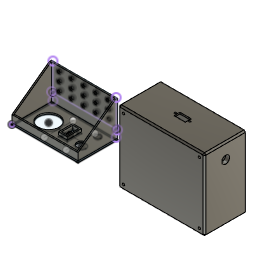
12v-socket-mounting-bracket_and_case (Autodesk Fusion 360 design; units mm, degrees)
Autodesk Fusion 360 part; units mm, degrees
sketch "Skizze1" plane through (0, 0, 0) normal (0, 0, 1) x (1, 0, 0) in component "Montagewinkel"
  line L0 (0, 0) -> (92, 0)
  line L1 (92, 0) -> (92, 55)
  line L2 (92, 55) -> (0, 55)
  line L3 (0, 55) -> (0, 0)
  line L4 (2, 2) -> (90, 2)
  line L5 (90, 2) -> (90, 53)
  line L6 (90, 53) -> (2, 53)
  line L7 (2, 53) -> (2, 2)
  line L8 (2, 53) -> (2, 55)
  line L9 (90, 53) -> (90, 55)
  line L10 (2, 2) -> (2, 0)
  line L11 (90, 2) -> (90, 0)
  circle A0 centre (23.5, 27.5) radius 14.5
  circle A1 centre (74.5, 22) radius 6
  circle A2 centre (74.5, 45) radius 4
  line L12 (38, 47) -> (38, 7) construction
  line L13 (68.5, 47) -> (68.5, 7) construction
  line L14 (68.5, 27.5) -> (38, 27.5) construction
  line L15 (57.325, 19.625) -> (49.175, 19.625)
  line L16 (49.175, 19.625) -> (49.175, 35.375)
  line L17 (49.175, 35.375) -> (57.325, 35.375)
  line L18 (57.325, 35.375) -> (57.325, 19.625)
  line L19 (57.325, 19.625) -> (49.175, 35.375) construction
  line L20 (49.175, 19.625) -> (57.325, 35.375) construction
  line L21 (59.325, 17.625) -> (47.175, 17.625)
  line L22 (47.175, 17.625) -> (47.175, 37.375)
  line L23 (47.175, 37.375) -> (59.325, 37.375)
  line L24 (59.325, 37.375) -> (59.325, 17.625)
  point P0 (53.25, 27.5)
  dimension "d1" = 92
  dimension "d2" = 55
  dimension "d4" = 29
  dimension "d5" = 23.5
  dimension "d6" = 27.5
  dimension "d7" = 12
  dimension "d8" = 22
  dimension "d9" = 17.5
  dimension "d10" = 8
  dimension "d11" = 10
  dimension "d12" = 17.5
  dimension "d13" = 27.5
  dimension "d14" = 8.15
  dimension "d15" = 15.75
  constraint horizontal L0
  constraint vertical L1
  constraint horizontal L2
  constraint vertical L3
  constraint coincident L0.start L3.end
  constraint coincident L2 L8.end
  constraint perpendicular L2 L8
  constraint coincident L2 L9.end
  constraint perpendicular L2 L9
  constraint coincident L0 L10.end
  constraint perpendicular L0 L10
  constraint coincident L0 L11.end
  constraint perpendicular L0 L11
  constraint vertical L12
  constraint tangent A0 L12
  constraint vertical L13
  constraint tangent A1 L13
  constraint coincident L13 L14.start
  constraint coincident L12 L14.end
  constraint perpendicular L12 L14
  constraint horizontal L15
  constraint perpendicular L15 L16
  constraint parallel L15 L17
  constraint parallel L16 L18
  constraint coincident L19 P0
  constraint coincident L20 P0
  constraint midpoint L14 P0
  measures "d1" distance of L0.start L0.end
  measures "d2" distance of L0.start L2.end
  measures "d4" diameter of A0
  measures "d5" distance of L3 A0.centre
  measures "d6" distance of L2 A0.centre
  measures "d7" diameter of A1
  measures "d8" distance of L0 A1.centre
  measures "d9" distance of L1 A1.centre
  measures "d10" diameter of A2
  measures "d11" distance of L2 A2.centre
  measures "d12" distance of L1 A2.centre
  measures "d13" distance of L2 L14
  measures "d14" distance of L16.end L17.end
  measures "d15" distance of L15.end L16.end
extrude "Extrusion1" add sketch "Skizze1" along normal blind 2 contours L4 L5 L6 L7 makes body 1 in component "Montagewinkel"
extrude "Extrusion3" add sketch "Skizze1" along normal blind 6 contours L21 L22 L23 L24 bodies 1 in component "Montagewinkel"
extrude "Extrusion4" add sketch "Skizze1" along normal blind 50 contours L0 L2 L3 L7 L8 L10 | L0 L1 L2 L5 L9 L11 | L2 L6 L8 L9 bodies 1 in component "Montagewinkel"
extrude "Extrusion5" add sketch "Skizze1" along normal blind 12 contours L0 L4 L10 L11 bodies 1 in component "Montagewinkel"
chamfer "Fase1" distance 52 distance2 38 2 edges at (1, 0, 50) (91, 0, 50) measured on face at (31.3333, 54.3333, 50) measured on face at (31.3333, 54.3333, 50) on bodies 1 in component "Montagewinkel"
chamfer "Fase2" distance 2 angle 45 3 edges at (46, 0, 0) (0, 27.5, 0) (92, 27.5, 0) on bodies 1 in component "Montagewinkel"
sketch "Skizze2" plane through (0, 55, 0) normal (0, 1, 0) x (-1, 0, 0) in component "Montagewinkel"
  line L0 (-92, 2) -> (-90, 0)
  line L1 (-90, 0) -> (-2, 0)
  line L2 (-2, 0) -> (0, 2)
  line L3 (0, 2) -> (0, 50)
  line L4 (0, 50) -> (-92, 50)
  line L5 (-92, 50) -> (-92, 2)
  line L6 (0, 12) -> (-2, 12)
  line L7 (-2, 12) -> (-90, 12)
  line L8 (-90, 12) -> (-92, 12)
  line L9 (-2, 2) -> (-2, 50)
  line L10 (-90, 2) -> (-90, 50)
  circle A0 centre (-80, 19) radius 1.8
  circle A1 centre (-63, 19) radius 1.8
  circle A2 centre (-80, 31) radius 1.8
  circle A3 centre (-63, 31) radius 1.8
  circle A4 centre (-46, 19) radius 1.8
  circle A5 centre (-29, 19) radius 1.8
  circle A6 centre (-12, 19) radius 1.8
  circle A7 centre (-46, 31) radius 1.8
  circle A8 centre (-29, 31) radius 1.8
  circle A9 centre (-12, 31) radius 1.8
  circle A10 centre (-80, 43) radius 1.8
  circle A11 centre (-63, 43) radius 1.8
  circle A12 centre (-46, 43) radius 1.8
  circle A13 centre (-29, 43) radius 1.8
  circle A14 centre (-12, 43) radius 1.8
  dimension "d30" = 3.6
  dimension "d31" = 10
  dimension "d32" = 7
  dimension "d36" = 68
  dimension "d37" = 24
  measures "d30" diameter of A0
  measures "d31" distance of L10 A0.centre
  measures "d32" distance of L7 A0.centre
extrude "Extrusion6" cut sketch "Skizze2" against normal blind 2 contours A0 | A1 | A2 | A3 | A4 | A5 | A6 | A7 | A8 | A9 | A10 | A11 | A12 | A13 | A14 bodies 1 in component "Montagewinkel"
sketch "Skizze1 (2)" plane through (0, 0, 0) normal (0, 0, 1) x (1, 0, 0) in component "Gehäuse"
  line L0 (0, 0) -> (120, 0)
  line L1 (120, 0) -> (120, 55)
  line L2 (120, 55) -> (0, 55)
  line L3 (0, 55) -> (0, 0)
  circle A0 centre (32.7, 27.5) radius 14.5
  circle A1 centre (93.3, 22) radius 6
  circle A2 centre (93.3, 45) radius 4
  line L4 (47.2, 47) -> (47.2, 7) construction
  line L5 (87.3, 47) -> (87.3, 7) construction
  line L6 (87.3, 27.5) -> (47.2, 27.5) construction
  line L7 (71.325, 19.625) -> (63.175, 19.625)
  line L8 (63.175, 19.625) -> (63.175, 35.375)
  line L9 (63.175, 35.375) -> (71.325, 35.375)
  line L10 (71.325, 35.375) -> (71.325, 19.625)
  line L11 (71.325, 19.625) -> (63.175, 35.375) construction
  line L12 (63.175, 19.625) -> (71.325, 35.375) construction
  line L13 (73.325, 17.625) -> (61.175, 17.625)
  line L14 (61.175, 17.625) -> (61.175, 37.375)
  line L15 (61.175, 37.375) -> (73.325, 37.375)
  line L16 (73.325, 37.375) -> (73.325, 17.625)
  point P0 (67.25, 27.5)
  dimension "d1_1" = 120
  dimension "d2_1" = 55
  dimension "d4_1" = 29
  dimension "d5_1" = 32.7
  dimension "d6_1" = 27.5
  dimension "d7_1" = 12
  dimension "d8_1" = 22
  dimension "d9_1" = 26.7
  dimension "d10_1" = 8
  dimension "d11_1" = 10
  dimension "d12_1" = 26.7
  dimension "d13_1" = 27.5
  dimension "d14_1" = 8.15
  dimension "d15_1" = 15.75
  constraint horizontal L0
  constraint vertical L1
  constraint horizontal L2
  constraint vertical L3
  constraint coincident L0.start L3.end
  constraint vertical L4
  constraint tangent A0 L4
  constraint vertical L5
  constraint tangent A1 L5
  constraint coincident L5 L6.start
  constraint coincident L4 L6.end
  constraint perpendicular L4 L6
  constraint horizontal L7
  constraint perpendicular L7 L8
  constraint parallel L7 L9
  constraint parallel L8 L10
  constraint coincident L11 P0
  constraint coincident L12 P0
  constraint midpoint L6 P0
  measures "d1_1" distance of L0.start L0.end
  measures "d2_1" distance of L0.start L2.end
  measures "d4_1" diameter of A0
  measures "d5_1" distance of L3 A0.centre
  measures "d6_1" distance of L2 A0.centre
  measures "d7_1" diameter of A1
  measures "d8_1" distance of L0 A1.centre
  measures "d9_1" distance of L1 A1.centre
  measures "d10_1" diameter of A2
  measures "d11_1" distance of L2 A2.centre
  measures "d12_1" distance of L1 A2.centre
  measures "d13_1" distance of L2 L6
  measures "d14_1" distance of L8.end L9.end
  measures "d15_1" distance of L7.end L8.end
extrude "Extrusion8" add sketch "Skizze1 (2)" along normal blind 100 separate body contours L0 L1 L2 L3 | A0 | A1 | A2 | L7 L8 L9 L10 | L13 L14 L15 L16 makes body 2 in component "Gehäuse"
shell "Schale1" thickness 2 removed faces 1 at (40, 0, 66.6667) on bodies 2 in component "Gehäuse"
chamfer "Fase4" distance 2 angle 45 4 edges at (120, 27.5, 100) (0, 27.5, 100) (0, 27.5, 0) (120, 27.5, 0) on bodies 2 in component "Gehäuse"
extrude "Extrusion9" cut sketch "Skizze1 (2)" along normal blind 2 contours A0 | A1 | A2 | L7 L8 L9 L10 bodies 2 in component "Gehäuse"
extrude "Extrusion10" add sketch "Skizze1 (2)" along normal blind 6 contours L13 L14 L15 L16 bodies 2 in component "Gehäuse"
sketch "Skizze4" plane through (0, 53, 0) normal (0, -1, 0) x (1, 0, 0) in component "Gehäuse"
  line L0 (2, 2) -> (118, 2)
  line L1 (118, 2) -> (118, 98)
  line L2 (118, 98) -> (2, 98)
  line L3 (2, 98) -> (2, 2)
  circle A0 centre (7.2, 92.8) radius 5.2
  circle A1 centre (7.2, 92.8) radius 1.25
  circle A2 centre (112.8, 92.8) radius 5.2
  circle A3 centre (112.8, 92.8) radius 1.25
  circle A4 centre (7.2, 7.2) radius 5.2
  circle A5 centre (7.2, 7.2) radius 1.25
  circle A6 centre (112.8, 7.2) radius 5.2
  circle A7 centre (112.8, 7.2) radius 1.25
  line L4 (12.4, 92.8) -> (12.4, 98)
  line L5 (7.2, 87.6) -> (2, 87.6)
  line L6 (107.6, 92.8) -> (107.6, 98)
  line L7 (112.8, 87.6) -> (118, 87.6)
  line L8 (12.4, 7.2) -> (12.4, 2)
  line L9 (7.2, 12.4) -> (2, 12.4)
  line L10 (112.8, 12.4) -> (118, 12.4)
  line L11 (107.6, 7.2) -> (107.6, 2)
  line L12 (13.5, 62) -> (7, 62)
  line L13 (7, 62) -> (7, 77)
  line L14 (7, 77) -> (13.5, 77)
  line L15 (13.5, 77) -> (13.5, 62)
  line L16 (13.5, 62) -> (7, 77) construction
  line L17 (7, 62) -> (13.5, 77) construction
  line L18 (55, 62) -> (48.5, 62)
  line L19 (48.5, 62) -> (48.5, 77)
  line L20 (48.5, 77) -> (55, 77)
  line L21 (55, 77) -> (55, 62)
  line L22 (55, 62) -> (48.5, 77) construction
  line L23 (48.5, 62) -> (55, 77) construction
  line L24 (113, 42) -> (106.5, 42)
  line L25 (106.5, 42) -> (106.5, 57)
  line L26 (106.5, 57) -> (113, 57)
  line L27 (113, 57) -> (113, 42)
  line L28 (113, 42) -> (106.5, 57) construction
  line L29 (106.5, 42) -> (113, 57) construction
  line L30 (71.5, 42) -> (65, 42)
  line L31 (65, 42) -> (65, 57)
  line L32 (65, 57) -> (71.5, 57)
  line L33 (71.5, 57) -> (71.5, 42)
  line L34 (71.5, 42) -> (65, 57) construction
  line L35 (65, 42) -> (71.5, 57) construction
  circle A8 centre (10.25, 69.5) radius 1.25
  circle A9 centre (68.25, 49.5) radius 1.25
  circle A10 centre (51.75, 69.5) radius 1.25
  circle A11 centre (109.75, 49.5) radius 1.25
  circle A12 centre (12, 22) radius 1.8
  line L36 (60, 98) -> (60, 2) construction
  circle A13 centre (108, 22) radius 1.8
  circle A14 centre (22, 88) radius 1.8
  line L37 (2, 98) -> (118, 98)
  line L38 (2, 2) -> (2, 98)
  circle A15 centre (98, 88) radius 1.8
  line L39 (118, 98) -> (118, 2)
  point P0 (10.25, 69.5)
  point P1 (51.75, 69.5)
  point P2 (109.75, 49.5)
  point P3 (68.25, 49.5)
  dimension "d68" = 5.2
  dimension "d69" = 2.5
  dimension "d70" = 5.2
  dimension "d71" = 2.5
  dimension "d72" = 5.2
  dimension "d73" = 2.5
  dimension "d74" = 5.2
  dimension "d75" = 2.5
  dimension "d78" = 6.5
  dimension "d79" = 15
  dimension "d80" = 5
  dimension "d81" = 60
  dimension "d82" = 15
  dimension "d83" = 6.5
  dimension "d84" = 48
  dimension "d85" = 60
  dimension "d86" = 15
  dimension "d87" = 6.5
  dimension "d88" = 5
  dimension "d89" = 6.5
  dimension "d90" = 15
  dimension "d91" = 48
  dimension "d92" = 40
  dimension "d93" = 40
  dimension "d94" = 2.5
  dimension "d95" = 2.5
  dimension "d96" = 2.5
  dimension "d97" = 2.5
  dimension "d162" = 3.6
  dimension "d163" = 20
  dimension "d164" = 10
  dimension "d165" = 3.6
  dimension "d166" = 10
  dimension "d167" = 20
  dimension "d168" = 3.6
  dimension "d169" = 10
  dimension "d170" = 20
  constraint tangent L2 A0
  constraint tangent L3 A0
  constraint concentric A0 A1
  constraint tangent L2 A2
  constraint tangent L1 A2
  constraint concentric A2 A3
  constraint tangent L3 A4
  constraint tangent L0 A4
  constraint concentric A4 A5
  constraint tangent L0 A6
  constraint tangent L1 A6
  constraint concentric A6 A7
  constraint coincident A0 L4.start
  constraint coincident L2 L4.end
  constraint tangent A0 L4
  constraint perpendicular L2 L4
  constraint coincident A0 L5.start
  constraint coincident L3 L5.end
  constraint tangent A0 L5
  constraint perpendicular L3 L5
  constraint coincident A2 L6.start
  constraint coincident L2 L6.end
  constraint tangent A2 L6
  constraint perpendicular L2 L6
  constraint coincident A2 L7.start
  constraint tangent A2 L7
  constraint perpendicular L6 L7
  constraint coincident A4 L8.start
  constraint coincident L0 L8.end
  constraint tangent A4 L8
  constraint perpendicular L0 L8
  constraint coincident A4 L9.start
  constraint coincident L3 L9.end
  constraint tangent A4 L9
  constraint perpendicular L3 L9
  constraint coincident A6 L10.start
  constraint coincident L1 L10.end
  constraint tangent A6 L10
  constraint perpendicular L1 L10
  constraint coincident A6 L11.start
  constraint coincident L0 L11.end
  constraint tangent A6 L11
  constraint perpendicular L0 L11
  constraint horizontal L12
  constraint perpendicular L12 L13
  constraint parallel L12 L14
  constraint parallel L13 L15
  constraint coincident L16 P0
  constraint coincident L17 P0
  constraint horizontal L18
  constraint perpendicular L18 L19
  constraint parallel L18 L20
  constraint parallel L19 L21
  constraint coincident L22 P1
  constraint coincident L23 P1
  constraint horizontal L24
  constraint perpendicular L24 L25
  constraint parallel L24 L26
  constraint parallel L25 L27
  constraint coincident L28 P2
  constraint coincident L29 P2
  constraint horizontal L30
  constraint perpendicular L30 L31
  constraint parallel L30 L32
  constraint parallel L31 L33
  constraint coincident L34 P3
  constraint coincident L35 P3
  constraint coincident P0 A8.centre
  constraint coincident P3 A9.centre
  constraint coincident P1 A10.centre
  constraint coincident P2 A11.centre
  constraint coincident L1 L7.end
  constraint midpoint L2 L36.start
  constraint midpoint L0 L36.end
  constraint symmetric A12 L36 A13
  measures "d68" radius of A0
  measures "d69" diameter of A1
  measures "d70" radius of A2
  measures "d71" diameter of A3
  measures "d72" radius of A4
  measures "d73" diameter of A5
  measures "d74" radius of A6
  measures "d75" diameter of A7
  measures "d78" distance of L13.end L14.end
  measures "d79" distance of L12.end L13.end
  measures "d80" distance of L3 L13
  measures "d81" distance of L0 L12
  measures "d82" distance of L18.end L19.end
  measures "d83" distance of L19.end L20.end
  measures "d84" distance of L13 L21
  measures "d85" distance of L0 L18
  measures "d86" distance of L24.end L25.end
  measures "d87" distance of L25.end L26.end
  measures "d88" distance of L1 L27
  measures "d89" distance of L31.end L32.end
  measures "d90" distance of L30.end L31.end
  measures "d91" distance of L27 L31
  measures "d92" distance of L0 L24
  measures "d93" distance of L0 L30
  measures "d94" diameter of A8
  measures "d95" diameter of A9
  measures "d96" diameter of A10
  measures "d97" diameter of A11
  measures "d162" diameter of A12
  measures "d163" distance of L0 A12.centre
  measures "d164" distance of L3 A12.centre
  measures "d165" diameter of A14
  measures "d166" distance of A14.centre L37
  measures "d167" distance of A14.centre L38
  measures "d168" diameter of A15
  measures "d169" distance of L2 A15.centre
  measures "d170" distance of A15.centre L39
extrude "Extrusion11" add sketch "Skizze4" along normal blind 53 contours L0 A4 L8 | L0 A6 L11 | L0 L3 A4 L38 | A4 | L0 L1 A6 L39 | A6 | L3 A4 L9 L38 | L1 A6 L10 L39 | L3 A0 L5 L38 | L1 A2 L7 L39 | L2 L3 A0 L37 L38 | A0 | L1 L2 A2 L37 L39 | A2 | L2 A0 L4 L37 | L2 A2 L6 L37 bodies 2 in component "Gehäuse"
extrude "Extrusion12" add sketch "Skizze4" along normal blind 15 contours L12 L13 L14 L15 | L18 L19 L20 L21 bodies 2 in component "Gehäuse"
extrude "Extrusion13" add sketch "Skizze4" along normal blind 20 contours L24 L25 L26 L27 | L30 L31 L32 L33 bodies 2 in component "Gehäuse"
extrude "Extrusion17" cut sketch "Skizze4" against normal blind 2 contours A12 | A13 | A14 | A15 bodies 2 in component "Gehäuse"
sketch "Skizze6" plane through (0, 0, 100) normal (0, 0, 1) x (-1, 0, 0) in component "Gehäuse"
  line L0 (-2, -55) -> (-2, 0)
  line L1 (-2, 0) -> (-118, 0)
  line L2 (-118, 0) -> (-118, -55)
  line L3 (-118, -55) -> (-2, -55)
  line L4 (-2, -55) -> (-118, 0) construction
  line L5 (-118, -55) -> (-2, 0) construction
  line L6 (-67.875, -23.425) -> (-52.125, -23.425)
  line L7 (-52.125, -23.425) -> (-52.125, -31.575)
  line L8 (-52.125, -31.575) -> (-67.875, -31.575)
  line L9 (-67.875, -31.575) -> (-67.875, -23.425)
  line L10 (-67.875, -23.425) -> (-52.125, -31.575) construction
  line L11 (-52.125, -23.425) -> (-67.875, -31.575) construction
  circle A0 centre (-49.75, -27.5) radius 1.25
  line L12 (-60, -31.575) -> (-60, -23.425) construction
  circle A1 centre (-70.25, -27.5) radius 1.25
  point P0 (-60, -27.5)
  dimension "d120" = 15.75
  dimension "d121" = 8.15
  dimension "d122" = 2.5
  dimension "d123" = 10.25
  dimension "d124" = 4.075
  constraint coincident L0.start L3.end
  constraint coincident L1.end L2.start
  constraint coincident L2.end L3.start
  constraint coincident L0.end L1.start
  constraint horizontal L6
  constraint perpendicular L6 L7
  constraint parallel L6 L8
  constraint parallel L7 L9
  constraint coincident L10 P0
  constraint coincident L11 P0
  constraint midpoint L4 P0
  constraint midpoint L8 L12.start
  constraint midpoint L6 L12.end
  constraint symmetric A0 L12 A1
  measures "d120" distance of L7.end L8.end
  measures "d121" distance of L6.end L7.end
  measures "d122" diameter of A0
  measures "d123" distance of P0 A0.centre
  measures "d124" distance of L6 A0.centre
extrude "Extrusion14" cut sketch "Skizze6" against normal blind 2 contours L6 L7 L8 L9 | A0 | A1 bodies 2 in component "Gehäuse"
sketch "Skizze7" plane through (120, 0, 0) normal (1, 0, 0) x (0, 1, 0) in component "Gehäuse"
  line L0 (0, 2) -> (55, 2)
  line L1 (55, 2) -> (55, 98)
  line L2 (55, 98) -> (0, 98)
  line L3 (0, 98) -> (0, 2)
  circle A0 centre (27.5, 78.8) radius 5.425
  line L4 (32.925, 73.375) -> (22.075, 73.375)
  line L5 (22.075, 73.375) -> (22.075, 84.225)
  line L6 (22.075, 84.225) -> (32.925, 84.225)
  line L7 (32.925, 84.225) -> (32.925, 73.375)
  line L8 (32.925, 73.375) -> (22.075, 84.225) construction
  line L9 (22.075, 73.375) -> (32.925, 84.225) construction
  line L10 (22.575, 84.225) -> (22.575, 73.375)
  circle A1 centre (27.5, 78.8) radius 7.425
  point P0 (27.5, 78.8)
  dimension "d148" = 10.85
  dimension "d149" = 27.5
  dimension "d150" = 19.2
  dimension "d151" = 10.85
  dimension "d152" = 10.85
  dimension "d153" = 4.925
  dimension "d158" = 2
  constraint horizontal L4
  constraint perpendicular L4 L5
  constraint parallel L4 L6
  constraint parallel L5 L7
  constraint coincident L8 P0
  constraint coincident L9 P0
  constraint coincident P0 A0.centre
  constraint coincident L6 L10.start
  constraint coincident L4 L10.end
  constraint perpendicular L4 L10
  measures "d148" diameter of A0
  measures "d149" distance of L1 P0
  measures "d150" distance of L2 P0
  measures "d151" distance of L5.end L6.end
  measures "d152" distance of L4.end L5.end
  measures "d153" distance of P0 L10
extrude "Extrusion15" cut sketch "Skizze7" against normal blind 2 contours A0 L10 picked at (25.8622, 77.1855) bodies 2 in component "Gehäuse"
extrude "Extrusion16" add sketch "Skizze7" against normal blind 5.5 contours A0 L4 L7 A1 | A0 L6 L7 A1 | L7 A1 | A0 L6 L10 | L6 A1 | A0 L4 L10 | L4 A1 | A0 L10 | A0 L5 L6 L10 A1 | A0 L4 L5 L10 A1 | L5 A1 picked at (22.4831, 79.3144) bodies 2 in component "Gehäuse"
draft "Entwurf5" angle 25 neutral plane through (0, 38, 0) pull (0, -1, 0) 1 faces at (55, 48, 72) on bodies 2 in component "Gehäuse"
draft "Entwurf6" angle 25 neutral plane through (0, 33, 0) pull (0, -1, 0) 1 faces at (65, 46.3333, 47) on bodies 2 in component "Gehäuse"
draft "Entwurf7" angle 25 neutral plane through (0, 38, 0) pull (0, -1, 0) 1 faces at (7, 48, 67) on bodies 2 in component "Gehäuse"
draft "Entwurf8" angle 25 neutral plane through (0, 33, 0) pull (0, -1, 0) 1 faces at (113, 46.3333, 52) on bodies 2 in component "Gehäuse"
sketch "Skizze1 (3)" plane through (0, 0, 0) normal (0, -1, 0) x (1, 0, 0) in component "Gehäusedeckel"
  circle A0 centre (262.8, 7.2) radius 1.25
  circle A1 centre (157.2, 92.8) radius 1.25
  circle A2 centre (157.2, 7.2) radius 1.25
  circle A3 centre (262.8, 92.8) radius 1.25
  line L0 (268, 0) -> (270, 2)
  line L1 (270, 2) -> (270, 98)
  line L2 (270, 98) -> (268, 100)
  line L3 (268, 100) -> (152, 100)
  line L4 (152, 100) -> (150, 98)
  line L5 (150, 98) -> (150, 2)
  line L6 (150, 2) -> (152, 0)
  line L7 (152, 0) -> (268, 0)
  line L8 (152, 12.4) -> (152, 87.6)
  line L9 (152, 87.6) -> (157.2, 87.6)
  arc A4 (157.2, 87.6) -> (162.4, 92.8) centre (157.2, 92.8) ccw
  line L10 (162.4, 92.8) -> (162.4, 98)
  line L11 (162.4, 98) -> (257.6, 98)
  line L12 (257.6, 98) -> (257.6, 92.8)
  arc A5 (257.6, 92.8) -> (262.8, 87.6) centre (262.8, 92.8) ccw
  line L13 (262.8, 87.6) -> (268, 87.6)
  line L14 (268, 87.6) -> (268, 12.4)
  line L15 (268, 12.4) -> (262.8, 12.4)
  arc A6 (262.8, 12.4) -> (257.6, 7.2) centre (262.8, 7.2) ccw
  line L16 (257.6, 7.2) -> (257.6, 2)
  line L17 (257.6, 2) -> (162.4, 2)
  line L18 (162.4, 2) -> (162.4, 7.2)
  arc A7 (162.4, 7.2) -> (157.2, 12.4) centre (157.2, 7.2) ccw
  line L19 (157.2, 12.4) -> (152, 12.4)
  circle A8 centre (157.2, 92.8) radius 1.6
  circle A9 centre (262.8, 92.8) radius 1.6
  circle A10 centre (262.8, 7.2) radius 1.6
  circle A11 centre (157.2, 7.2) radius 1.6
  line L20 (162.6, 92.8) -> (162.6, 97.8)
  line L21 (162.6, 97.8) -> (257.4, 97.8)
  line L22 (257.4, 97.8) -> (257.4, 92.8)
  arc A12 (257.4, 92.8) -> (262.8, 87.4) centre (262.8, 92.8) ccw
  line L23 (262.8, 87.4) -> (267.8, 87.4)
  line L24 (267.8, 87.4) -> (267.8, 12.6)
  line L25 (267.8, 12.6) -> (262.8, 12.6)
  arc A13 (262.8, 12.6) -> (257.4, 7.2) centre (262.8, 7.2) ccw
  line L26 (257.4, 7.2) -> (257.4, 2.2)
  line L27 (257.4, 2.2) -> (162.6, 2.2)
  line L28 (162.6, 2.2) -> (162.6, 7.2)
  arc A14 (162.6, 7.2) -> (157.2, 12.6) centre (157.2, 7.2) ccw
  line L29 (157.2, 12.6) -> (152.2, 12.6)
  line L30 (152.2, 12.6) -> (152.2, 87.4)
  line L31 (152.2, 87.4) -> (157.2, 87.4)
  arc A15 (157.2, 87.4) -> (162.6, 92.8) centre (157.2, 92.8) ccw
  line L32 (164.6, 95.8) -> (255.4, 95.8)
  line L33 (255.4, 95.8) -> (255.4, 92.8)
  arc A16 (255.4, 92.8) -> (262.8, 85.4) centre (262.8, 92.8) ccw
  line L34 (262.8, 85.4) -> (265.8, 85.4)
  line L35 (265.8, 85.4) -> (265.8, 14.6)
  line L36 (265.8, 14.6) -> (262.8, 14.6)
  arc A17 (262.8, 14.6) -> (255.4, 7.2) centre (262.8, 7.2) ccw
  line L37 (255.4, 7.2) -> (255.4, 4.2)
  line L38 (255.4, 4.2) -> (164.6, 4.2)
  line L39 (164.6, 4.2) -> (164.6, 7.2)
  arc A18 (164.6, 7.2) -> (157.2, 14.6) centre (157.2, 7.2) ccw
  line L40 (157.2, 14.6) -> (154.2, 14.6)
  line L41 (154.2, 14.6) -> (154.2, 85.4)
  line L42 (154.2, 85.4) -> (157.2, 85.4)
  arc A19 (157.2, 85.4) -> (164.6, 92.8) centre (157.2, 92.8) ccw
  line L43 (164.6, 92.8) -> (164.6, 95.8)
  dimension "d137" = 3.2
  dimension "d138" = 3.2
  dimension "d139" = 3.2
  dimension "d140" = 3.2
  dimension "d141" = 0.2
  dimension "d143" = 2.2
  constraint concentric A1 A8
  constraint concentric A3 A9
  constraint concentric A0 A10
  constraint concentric A2 A11
  measures "d137" diameter of A8
  measures "d138" diameter of A9
  measures "d139" diameter of A10
  measures "d140" diameter of A11
extrude "Extrusion1'" add sketch "Skizze1 (3)" along normal blind 2 separate body contours L0 L1 L2 L3 L4 L5 L6 L7 | L8 L9 A4 L10 L11 L12 A5 L13 L14 L15 A6 L16 L17 L18 A7 L19 | L20 L21 L22 A12 L23 L24 L25 A13 L26 L27 L28 A14 L29 L30 L31 A15 | L32 L33 A16 L34 L35 L36 A17 L37 L38 L39 A18 L40 L41 L42 A19 L43 makes body 3 in component "Gehäusedeckel"
extrude "Extrusion2" add sketch "Skizze1 (3)" against normal blind 2 contours L20 L21 L22 A12 L23 L24 L25 A13 L26 L27 L28 A14 L29 L30 L31 A15 bodies 3 in component "Gehäusedeckel"
chamfer "Fase1'" distance 2 angle 45 8 edges at (210, -2, 100) (269, -2, 99) (270, -2, 50) (269, -2, 1) (210, -2, 0) (151, -2, 1) (150, -2, 50) (151, -2, 99) on bodies 3 in component "Gehäusedeckel"
component "Montagewinkel" placed x (1, 0, 0) y (0, 1, 0) z (0, 0, 1) at (0, 0, 0)
component "Gehäuse" placed x (1, 0, 0) y (0, 1, 0) z (0, 0, 1) at (150, 0, 0)
component "Gehäusedeckel" placed x (1, 0, 0) y (0, 1, 0) z (0, 0, 1) at (0, 0, 0)
equation "d1 = bracket_width"
equation "d2 = case_depth"
equation "d3 = -wall_strength"
equation "d4 = socket_cutout_12v"
equation "d5 = socket_diameter_12v / 2 + component_gap"
equation "d6 = case_depth / 2"
equation "d7 = switch_cutout_diameter"
equation "d8 = switch_depth / 2 + component_gap"
equation "d9 = switch_width / 2 + component_gap"
equation "d10 = led_cutout_diameter"
equation "d11 = led_diameter / 2 + component_gap"
equation "d12 = switch_width / 2 + component_gap"
equation "d13 = case_depth / 2"
equation "d14 = xt60_plug_width"
equation "d15 = xt60_plug_length"
equation "d16 = -wall_strength"
equation "d1_1 = case_width"
equation "d2_1 = case_depth"
equation "d4_1 = socket_cutout_12v"
equation "d5_1 = ( socket_diameter_12v / 2 ) + case_min_component_offset"
equation "d6_1 = case_depth / 2"
equation "d7_1 = switch_cutout_diameter"
equation "d8_1 = switch_depth / 2 + component_gap"
equation "d9_1 = switch_width / 2 + case_min_component_offset"
equation "d10_1 = led_cutout_diameter"
equation "d11_1 = led_diameter / 2 + component_gap"
equation "d12_1 = switch_width / 2 + case_min_component_offset"
equation "d13_1 = case_depth / 2"
equation "d14_1 = xt60_plug_width"
equation "d15_1 = xt60_plug_length"
equation "d16_1 = -wall_strength"
equation "d44 = case_length"
equation "wall_strength = 2 mm"
equation "d47 = wall_strength"
equation "d49 = wall_strength"
equation "bus_bar_width = 15 mm"
equation "case_length = 100 mm"
equation "case_width = 120 mm"
equation "case_depth = 55 mm"
equation "socket_cutout_12v = 29 mm"
equation "socket_diameter_12v = 37 mm"
equation "component_gap = 5 mm"
equation "switch_width = 25 mm"
equation "switch_depth = 34 mm"
equation "xt60_plug_width = 8.15 mm"
equation "xt60_plug_length = 15.75 mm"
equation "led_diameter = 10 mm"
equation "led_cutout_diameter = 8 mm"
equation "switch_cutout_diameter = 12 mm"
equation "case_tap_diameter = 2.5 mm"
equation "d68 = lid_screw_dia + wall_strength"
equation "d69 = case_tap_diameter"
equation "d70 = lid_screw_dia + wall_strength"
equation "d71 = case_tap_diameter"
equation "d72 = lid_screw_dia + wall_strength"
equation "d73 = case_tap_diameter"
equation "d74 = lid_screw_dia + wall_strength"
equation "d75 = case_tap_diameter"
equation "lid_screw_dia = 3.2 mm"
equation "bus_bar_length = round(case_width * 0.4)"
equation "d78 = case_tap_diameter + 2 * wall_strength"
equation "d79 = bus_bar_width"
equation "d80 = component_gap"
equation "d81 = case_length / 2 + 2 * component_gap"
equation "d82 = bus_bar_width"
equation "d83 = case_tap_diameter + 2 * wall_strength"
equation "d84 = bus_bar_length"
equation "d85 = case_length / 2 + 2 * component_gap"
equation "d86 = bus_bar_width"
equation "d87 = case_tap_diameter + 2 * wall_strength"
equation "d88 = component_gap"
equation "d89 = case_tap_diameter + 2 * wall_strength"
equation "d90 = bus_bar_width"
equation "d91 = bus_bar_length"
equation "d92 = case_length / 2 - 2 * component_gap"
equation "d93 = case_length / 2 - 2 * component_gap"
equation "d94 = case_tap_diameter"
equation "d95 = case_tap_diameter"
equation "d96 = case_tap_diameter"
equation "d97 = case_tap_diameter"
equation "d98 = case_depth - wall_strength"
equation "d100 = component_gap * 3"
equation "d102 = component_gap * 4"
equation "bus_bar_support_angle = 25 deg"
equation "bracket_width = 92 mm"
equation "case_min_component_offset = 3 * wall_strength + lid_screw_dia + component_gap"
equation "xt60_socket_hole_spacing = 20.5 mm"
equation "d120 = xt60_plug_length"
equation "d121 = xt60_plug_width"
equation "d122 = case_tap_diameter"
equation "d123 = xt60_socket_hole_spacing / 2"
equation "d124 = xt60_plug_width / 2"
equation "d125 = -wall_strength"
equation "d127 = bus_bar_support_angle"
equation "d129 = bus_bar_support_angle"
equation "d131 = bus_bar_support_angle"
equation "d133 = bus_bar_support_angle"
equation "d135 = wall_strength"
equation "d137 = lid_screw_dia"
equation "d138 = lid_screw_dia"
equation "d139 = lid_screw_dia"
equation "d140 = lid_screw_dia"
equation "d141 = lid_gap"
equation "lid_gap = 0.2 mm"
equation "d143 = wall_strength + lid_gap"
equation "d144 = -wall_strength"
equation "fuse_hole_diameter = 10.85 mm"
equation "d148 = fuse_hole_diameter"
equation "d149 = case_depth / 2"
equation "d150 = case_min_component_offset + component_gap"
equation "d151 = fuse_hole_diameter"
equation "d152 = fuse_hole_diameter"
equation "d153 = fuse_hole_diameter_short / 2"
equation "d154 = -wall_strength"
equation "fuse_hole_diameter_short = 9.85 mm"
equation "fuse_hole_spacing = 5.5 mm - wall_strength"
equation "d158 = wall_strength"
equation "d159 = -( wall_strength + fuse_hole_spacing )"
equation "mounting_screw_hole = 3.6 mm"
equation "d162 = mounting_screw_hole"
equation "d163 = component_gap * 4"
equation "d164 = component_gap * 2"
equation "d165 = mounting_screw_hole"
equation "d166 = 2 * component_gap"
equation "d167 = 4 * component_gap"
equation "d168 = mounting_screw_hole"
equation "d169 = 2 * component_gap"
equation "d170 = 4 * component_gap"
equation "d171 = -wall_strength"
named bodies: "Montagewinkel"
